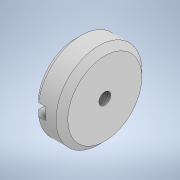
# Autodesk Inventor part: 711133
Saved by Autodesk Inventor 2022 (Build 260153000, 153)
## iProperties
Created: 2021-10-22
Part Number: 711133
Material: Типовые
Document SubType Name: Modeling
Designer: RaNSiD
Density: 1 g/cm^3
Appearance: По умолчанию
Author: RaNSiD
Autodesk Inventor part; units mm, degrees
ref_plane "YZ Plane" through (0, 0, 0) normal (1, 0, 0) x (0, 1, 0)
ref_plane "XZ Plane" through (0, 0, 0) normal (0, 1, 0) x (-1, 0, 0)
ref_plane "XY Plane" through (0, 0, 0) normal (0, 0, 1) x (1, 0, 0)
sketch "Эскиз4" plane through (0, 0, 0) normal (0, 0, 1) x (1, 0, 0)
  line L0 (0, 0) -> (20, 0)
  line L1 (20, 0) -> (20, 25)
  line L2 (16, 29) -> (4, 29)
  line L3 (0, 25) -> (0, 0)
  line L4 (4, 29) -> (0, 25)
  line L5 (16, 29) -> (20, 25)
  point P0 (20, 29)
  point P1 (0, 29)
  dimension "d20" = 20
  dimension "d21" = 29
  dimension "d22" = 4
  dimension "d23" = 4
  dimension "d24" = 4
  dimension "d25" = 4
  constraints: 12 end point, 4 point on line, 2 parallel, 1 horizontal, 1 perpendicular
  measures "d20" distance of point (0, 29) point (20, 29)
  measures "d21" distance of point (20, 29) L0.end
  measures "d22" distance of L2.end point (0, 29)
  measures "d23" distance of L3.start point (0, 29)
  measures "d24" distance of L2.start point (20, 29)
  measures "d25" distance of L1.end point (20, 29)
revolve "Вращение3" add sketch "Эскиз4" angle 360 about axis through (0, 0, 0) along (1, 0, 0)
sketch "Эскиз5" plane through (0, 0, 0) normal (0, 0, 1) x (1, 0, 0)
  line L0 (0, 4) -> (9, 4)
  line L1 (9, 4) -> (9, -4)
  line L2 (9, -4) -> (0, -4)
  line L3 (0, -4) -> (0, 4)
  point P0 (0, 0)
  point P1 (0, 0)
  dimension "d27" = 9
  dimension "d28" = 8
  constraints: 8 end point, 2 coincident, 2 parallel, 1 horizontal, 1 midpoint, 1 perpendicular
  measures "d27" distance of L1.end L2.end
  measures "d28" distance of L0.end L1.end
extrude "Выдавливание2" cut sketch "Эскиз5" along normal through all both and the other way through all
sketch "Эскиз6" plane through (20, 0, 0) normal (1, 0, 0) x (0, 0, -1)
  point P0 (0, 0)
  point P1 (0, 0)
  constraints: 1 coincident
hole "Отверстие1" at (20, 0, 0) direction (-1, 0, 0) diameter 8 depth 6
sketch "Эскиз7" plane through (14, 0, 0) normal (1, 0, 0) x (0, 0, -1)
  circle A0 centre (0, 0) radius 4.5
  dimension "d38" = 9
  constraints: 1 centre point, 1 coincident
  measures "d38" diameter of A0
extrude "Выдавливание3" cut sketch "Эскиз7" against normal blind 0.5
thread "Резьба3" size "M8x1.25" class "6H" standard "ANSI Metric M Profile" full length
equation "\"d23\" = d22"
equation "\"d24\" = d22"
equation "\"d25\" = d24"
